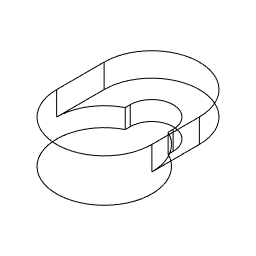
rev2-complete (Autodesk Fusion 360 archive; units mm, degrees)
design "Keyhole"
Autodesk Fusion 360 part; units mm, degrees
note: some values were not read from the file. Set by a fixed rule: which sketch regions a step uses.
sketch "Sketch6" plane through (0, 0, 0) normal (0, 1, 0) x (1, 0, 0)
  line L0 (5, 0) -> (5, -5)
  line L1 (-5, -5) -> (-5, 0)
  arc A0 (5, 0) -> (-5, 0) centre (0, 0) ccw
  arc A1 (-5, -5) -> (5, -5) centre (0, -5) ccw
  constraint vertical L0
  constraint vertical L1
extrude "Extrude4" add sketch "Sketch6" along normal blind 2.5
sketch "Sketch8" plane through (0, 2.5, 0) normal (0, 1, 0) x (-1, 0, 0)
  arc A0 (-5, 0) -> (5, 0) centre (0, 0) ccw
  line L0 (5, 0) -> (5, 5)
  arc A1 (5, 5) -> (-5, 5) centre (0, 5) ccw
  line L1 (-5, 5) -> (-5, 0)
  line L2 (-2.2505, 0.0027) -> (-2.2505, 0.5351)
  line L3 (2.25, 0.5349) -> (2.25, 0.0027)
  arc A2 (-2.25, 0.0027) -> (2.25, 0.0027) centre (0, 0) ccw
  arc A3 (2.25, 0.5349) -> (-2.2505, 0.5351) centre (0, 5) ccw
  line L4 (-2.25, 0.0027) -> (-2.2505, 0.0027)
  dimension "d20" = 4.5
  constraint concentric A0 A2
  constraint concentric A1 A3
  constraint coincident A1.end A3
  constraint vertical L2
  constraint vertical L3
  measures "d20" diameter of A2
extrude "Extrude6" add sketch "Sketch8" along normal blind 2 contours A1 L2 L3 A2 A3
move_body "Move3" bodies 1 to x (-0.999999, 0, 0.001644) y (0, -1, 0) z (0.001644, 0, 0.999999) at (-0.0082, 0, 0)
sketch "Sketch7" plane through (0, 2.5, 0) normal (0, 1, 0) x (-1, 0, 0)
  arc A0 (-5, 0) -> (5, 0) centre (0, 0) ccw
  line L0 (5, 0) -> (5, 5)
  arc A1 (5, 5) -> (-5, 5) centre (0, 5) ccw
  line L1 (-5, 5) -> (-5, 0)
  line L2 (-2.5, 5.5) -> (-2.5, 4.3301)
  line L3 (2.5, 4.3301) -> (2.5, 5.5)
  arc A2 (2.5, 5.5) -> (-2.5, 5.5) centre (0, 5.5) ccw
  arc A3 (-2.5, 4.3301) -> (2.5, 4.3301) centre (0, 0) ccw
  constraint coincident A0.centre A3.centre
  constraint coincident A0.start A3
  constraint vertical L2
  constraint vertical L3
extrude "Extrude5" [suppressed]
sketch "Sketch1" plane through (0, 0, 0) normal (0, 1, 0) x (1, 0, 0)
  line L0 (2.2439, 7.1121) -> (2.25, 7.1121)
  line L1 (2.25, 7.1121) -> (2.25, 4.4651)
  line L2 (-2.25, 4.4652) -> (-2.25, 7.1121)
  arc A0 (2.2439, 7.1121) -> (-2.25, 6.8778) centre (-0.003, 6.9949) ccw
  arc A1 (-2.25, 4.4652) -> (2.25, 4.4651) centre (0, 0) ccw
  dimension "d1" = 4.5
  dimension "d2" = 4.5
  dimension "d15" = 6.9949
  constraint coincident A1.centre origin
  constraint horizontal L0
  constraint vertical L1
  constraint vertical L2
  constraint coincident L2.end A0
  constraint coincident L2 A0.end
  measures "d1" diameter of A0
  measures "d2" distance of L2.end L0.end
  measures "d15" distance of A1.centre A0.centre
extrude "Extrude1" [suppressed]
sketch "Sketch4" plane through (0, 2.5, 0) normal (0, 1, 0) x (-1, 0, 0)
  line L0 (2.25, -7.1121) -> (2.25, -4.4652)
  arc A0 (2.25, -4.4652) -> (-2.25, -4.4651) centre (0, 0) ccw
  line L1 (-2.25, -4.4651) -> (-2.25, -7.1121)
  line L2 (-2.25, -7.1121) -> (-2.2439, -7.1121)
  arc A1 (-2.2439, -7.1121) -> (2.25, -7.1121) centre (0.003, -6.9949) ccw
  line L3 (-4.9966, -7.1563) -> (-4.9974, -7.1563)
  line L4 (-4.9974, -7.1563) -> (-4.9974, -0.026)
  line L5 (4.9999, -0.026) -> (5.0026, -0.026)
  line L6 (5.0026, -0.026) -> (5.0026, -7.1563)
  arc A2 (-4.9966, -7.1563) -> (5.0026, -7.0336) centre (0.003, -7.0949) ccw
  arc A3 (4.9999, -0.026) -> (-4.9974, -0.1627) centre (0, 0) ccw
  dimension "d7" = 10
  dimension "d8" = 10
  constraint coincident A0.centre A3.centre
  constraint horizontal L3
  constraint vertical L4
  constraint horizontal L5
  constraint vertical L6
  constraint coincident L6.end A2
  constraint coincident L6 A2.end
  constraint coincident L4 A3.end
  measures "d7" diameter of A2
  measures "d8" distance of L6.end L3.end
extrude "Extrude3" [suppressed]
move_body "Move1" [suppressed]
move_body "Move2" [suppressed]

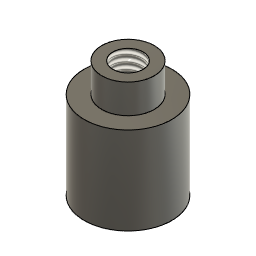
design "Standoffs"
Autodesk Fusion 360 part; units mm, degrees
sketch "Sketch1" plane through (0, 0, 0) normal (0, 1, 0) x (1, 0, 0)
  circle A0 centre (0, 0) radius 3
  constraint coincident A0.centre origin
extrude "Extrude1" add sketch "Sketch1" along normal blind 6
sketch "Sketch2" plane through (0, 6, 0) normal (0, 1, 0) x (-1, 0, 0)
  circle A0 centre (0, 0) radius 3
  circle A1 centre (0, 0) radius 1.8
  constraint concentric A0 A1
extrude "Extrude2" add sketch "Sketch2" along normal blind 2 contours A1
hole "Hole1" at (0, 8, 0) direction (0, -1, 0) diameter 2.076 depth 6 tip angle 118
thread "Thread1" "ISO Metric profile 2.5 M2.5x0.45 6H"
